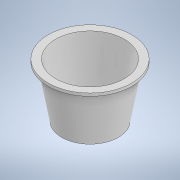
# Autodesk Inventor part: pingPongHolder 1-14
Saved by Autodesk Inventor 2020 (Build 240168000, 168)
## iProperties
Created: 2020-01-15
Part Number: pingPongHolder 1-14
Material: Generic
Document SubType Name: Modeling
Designer: akend
Density: 1 g/cm^3
Appearance: Default
Author: akend
Autodesk Inventor part; units mm, degrees
ref_plane "YZ Plane" through (0, 0, 0) normal (1, 0, 0) x (0, 1, 0)
ref_plane "XZ Plane" through (0, 0, 0) normal (0, 1, 0) x (-1, 0, 0)
ref_plane "XY Plane" through (0, 0, 0) normal (0, 0, 1) x (1, 0, 0)
sketch "Sketch1" plane through (0, 0, 0) normal (1, 0, 0) x (0, 1, 0)
  line L0 (0, 0) -> (-2.5, 0)
  line L1 (-2.5, 0) -> (-2.5, 22)
  line L2 (-2.5, 22) -> (0, 22)
  line L3 (0, 22) -> (0, 0)
  line L4 (0, 22) -> (44.3163, 29.8142)
  line L5 (0, 22) -> (45, 22) construction
  line L6 (44.3163, 29.8142) -> (43.7954, 32.7685)
  line L7 (43.7954, 32.7685) -> (-2.5, 24.6054)
  line L8 (-2.5, 24.6054) -> (-2.5, 22)
  line L9 (44.3163, 29.8142) -> (44.3163, 36.3142)
  line L10 (44.3163, 36.3142) -> (41.8163, 36.3142)
  line L11 (41.8163, 36.3142) -> (41.8163, 32.4195)
  line L12 (0, 0) -> (7.1877, 0)
  dimension "d0" = 2.5
  dimension "d1" = 22
  dimension "d2" = 45
  dimension "d3" = 10
  dimension "d4" = 6.5
  dimension "d5" = 2.5
  constraints: 26 end point, 4 perpendicular, 3 horizontal, 2 parallel, 2 vertical, 1 equal length, 1 point on line
  measures "d0" distance of L1.end L2.end
  measures "d1" distance of L0.end L1.end
  measures "d2" distance of L2.end L4.end
  measures "d3" angle of L5 L4
  measures "d4" distance of L4.end L9.end
  measures "d5" distance of L9.end L10.end
revolve "Revolution1" add sketch "Sketch1" angle 360 about axis through (0, 0, 0) along (0, 1, 0)
body "Solid1"
